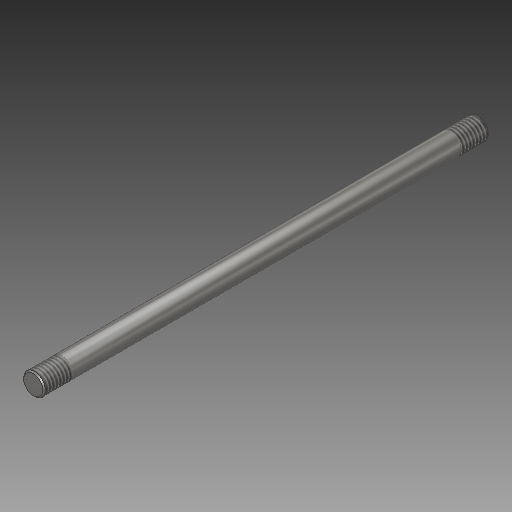
# Autodesk Inventor part: MecanumShaft
Saved by Autodesk Inventor 2018 (Build 220112000, 112)
## iProperties
Created: 2017-08-22
Part Number: MecanumShaft
Material: Steel, Carbon
Document SubType Name: Modeling
Designer: P136265
Density: 7.85 g/cm^3
Appearance: Semi-Polished
Mass: 64.2699 g
Surface Area: 41.8179 cm^2
Volume: 8.18725 cm^3
Author: P136265
Autodesk Inventor part; units mm, degrees
ref_plane "YZ Plane" through (0, 0, 0) normal (1, 0, 0) x (0, 1, 0)
ref_plane "XZ Plane" through (0, 0, 0) normal (0, 1, 0) x (-1, 0, 0)
ref_plane "XY Plane" through (0, 0, 0) normal (0, 0, 1) x (1, 0, 0)
sketch "Sketch1" plane through (0, 0, 0) normal (0, 0, 1) x (1, 0, 0)
  circle A0 centre (0, 0) radius 4
  dimension "d0" = 8
  constraints: 1 centre point, 1 coincident
  measures "d0" diameter of A0
extrude "Extrusion1" add sketch "Sketch1" along normal mid plane 163
chamfer "Chamfer1" distance 0.5 angle 45 2 edges at (-4, 0, 81.5) (-4, 0, -81.5)
thread "Thread1" size "M8x1.25" class "6g" standard "ANSI Metric M Profile" length 10
thread "Thread2" size "M8x1.25" class "6g" standard "ANSI Metric M Profile" length 10
body "Solid1"
